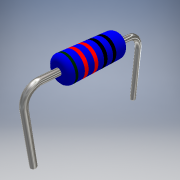
# Autodesk Inventor part: Resistor
Saved by Autodesk Inventor 2018 (Build 220112000, 112)
## iProperties
Created: 2021-02-04
Part Number: Resistor
Material: Všeobecné
Document SubType Name: Modeling
Designer: Jozko Mrkvicka
Density: 1 g/cm^3
Appearance: Výchozí
Author: Jozko Mrkvicka
Autodesk Inventor part; units mm, degrees
ref_plane "YZ Plane" through (0, 0, 0) normal (1, 0, 0) x (0, 1, 0)
ref_plane "XY Plane" through (0, 0, 0) normal (0, 0, 1) x (1, 0, 0)
sketch "Náčrt1" plane through (0, 0, 0) normal (0, 1, 0) x (-1, 0, 0)
  circle A0 centre (0, 0) radius 1.27
  dimension "d0" = 2.54
  constraints: 1 centre point, 1 coincident
  measures "d0" diameter of A0
extrude "Vysunutí1" add sketch "Náčrt1" along normal blind 6.35
sketch "Náčrt2" plane through (0, 0, 0) normal (1, 0, 0) x (0, 1, 0)
  point P0 (0, 0)
sketch "Náčrt3" plane through (0, 0, 0) normal (1, 0, 0) x (0, 1, 0)
  line L0 (0, 1.27) -> (0, -1.27) projected
  line L1 (6.35, -1.27) -> (6.35, 1.27) projected
  line L2 (0, 1.27) -> (6.35, 1.27)
  line L3 (0, 0) -> (-1.5873, 0)
  arc A0 (-1.5873, 0) -> (-3.1755, -1.589) centre (-1.5873, -1.5882) ccw
  arc A1 (9.53, -1.589) -> (7.9406, 0) centre (7.941, -1.589) ccw
  line L4 (9.53, -1.589) -> (9.53, -7.6277)
  line L5 (-3.1755, -1.589) -> (-3.1755, -7.6277)
  line L6 (7.9406, 0) -> (6.35, 0)
  point P0 (3.175, 1.27)
  point P1 (-3.1747, -3.1763)
  point P2 (9.5308, -3.1763)
  point P3 (0, -3.1763)
  point P4 (6.3512, -3.178)
  constraints: 10 end point, 4 point on circle, 2 centre point, 2 coincident, 2 horizontal, 2 midpoint, 2 vertical
sketch "Náčrt4" plane through (0, 0, 0) normal (0, -1, 0) x (1, 0, 0)
  circle A0 centre (0, 0) radius 1.27 projected
  circle A1 centre (0, 0) radius 0.3232
  constraints: 1 centre point, 1 coincident
sketch "Náčrt5" plane through (0, 6.35, 0) normal (0, 1, 0) x (1, 0, 0)
  circle A0 centre (0, 0) radius 1.27 projected
  circle A1 centre (0, 0) radius 0.3148
  constraints: 1 centre point, 1 coincident
sweep "Tažení1" add profiles "Náčrt4" path "Náčrt3" path curves L3 A0 L5 contours A1
sweep "Tažení2" add profiles "Náčrt5" path "Náčrt3" path curves L6 A1 L4 contours A1
fillet "Zaoblení1" radius 0.254 2 edges at (-0.3232, -3.1755, -7.6277) (-0.3148, 9.53, -7.6277)
fillet "Zaoblení2" radius 0.508 2 edges at (1.27, 0, 0) (1.27, 6.35, 0)
ref_plane "Pracovní rovina8" through (0, 4.445, 0) normal (0, 1, 0) x (-1, 0, 0)
ref_plane "Pracovní rovina7" through (0, 3.81, 0) normal (0, 1, 0) x (-1, 0, 0)
ref_plane "Pracovní rovina9" through (0, 4.826, 0) normal (0, 1, 0) x (-1, 0, 0)
split_face "Rozdělit1"
split_face "Rozdělit2"
split_face "Rozdělit3"
split_face "Rozdělit4"
split_face "Rozdělit5"
split_face "Rozdělit6"
split_face "Rozdělit7"
split_face "Rozdělit8"
split_face "Rozdělit9"
ref_plane "Pracovní rovina1" through (0, 0.762, 0) normal (0, 1, 0) x (-1, 0, 0)
ref_plane "Pracovní rovina2" through (0, 1.397, 0) normal (0, 1, 0) x (-1, 0, 0)
ref_plane "Pracovní rovina3" through (0, 1.778, 0) normal (0, 1, 0) x (-1, 0, 0)
ref_plane "Pracovní rovina4" through (0, 2.413, 0) normal (0, 1, 0) x (-1, 0, 0)
ref_plane "Pracovní rovina5" through (0, 2.794, 0) normal (0, 1, 0) x (-1, 0, 0)
ref_plane "Pracovní rovina6" through (0, 3.429, 0) normal (0, 1, 0) x (-1, 0, 0)
